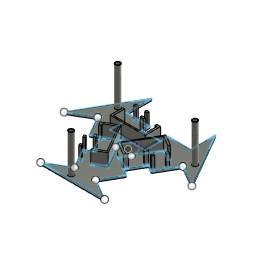
Bottom5 v3 (Autodesk Fusion 360 design; units mm, degrees)
Autodesk Fusion 360 part; units mm, degrees
sketch "草图1" plane through (0, 0, 0) normal (0, 1, 0) x (1, 0, 0)
  line L0 (0, 0) -> (6, 0)
  line L1 (6, 0) -> (6, 9.5)
  line L2 (0, 0) -> (-18.5, 0)
  line L3 (-18.5, 0) -> (-18.5, 9)
  line L4 (6, 9.5) -> (4.5, 9.5)
  line L5 (4.5, 9.5) -> (4.5, 11)
  line L6 (4.5, 11) -> (6, 11)
  line L7 (6, 11) -> (7.5, 11)
  line L8 (7.5, 11) -> (7.5, -1)
  line L9 (7.5, -1) -> (-20, -1)
  line L10 (-20, -1) -> (-20, 9)
  line L11 (-20, 9) -> (-18.5, 9)
  line L12 (-7, 11) -> (-7, 9.5)
  line L13 (-7, 9.5) -> (-4.5, 9.5)
  line L14 (-4.5, 9.5) -> (-4.5, 11)
  line L15 (-4.5, 11) -> (-7, 11)
  line L16 (-15.5, 15) -> (-17.5, 15)
  line L17 (-17.5, 15) -> (-17.5, 16.5)
  line L18 (-17.5, 16.5) -> (-15.5, 16.5)
  line L19 (-15.5, 16.5) -> (-15.5, 15)
  line L20 (-9, 15) -> (-7, 15)
  line L21 (-7, 15) -> (-7, 16.5)
  line L22 (-7, 16.5) -> (-9, 16.5)
  line L23 (-9, 16.5) -> (-9, 15)
  line L24 (4.8038, -27.3205) -> (-3.8564, -32.3205)
  line L25 (-19.3385, -9.5048) -> (-8.9462, -3.5048)
  line L26 (-17.8385, -12.1029) -> (-18.5885, -10.8038)
  line L27 (-6.0622, -10.5) -> (3.1878, -26.5215)
  line L28 (-8.9462, -3.5048) -> (4.8038, -27.3205)
  line L29 (-9.0622, -5.3038) -> (-17.2894, -10.0538)
  line L30 (-12.0394, -19.1471) -> (-13.3385, -19.8971)
  line L31 (-11.3026, -31.4234) -> (-10.3026, -33.1554)
  line L32 (-13.3385, -19.8971) -> (-12.0885, -22.0622)
  line L33 (-15.5526, -24.0622) -> (-16.8516, -24.8122)
  line L34 (3.1878, -26.5215) -> (-4.6064, -31.0215)
  line L35 (-16.8516, -24.8122) -> (-15.8516, -26.5442)
  line L36 (-15.8516, -26.5442) -> (-14.5526, -25.7942)
  line L37 (-6.0622, -10.5) -> (-9.0622, -5.3038)
  line L38 (-12.6016, -32.1734) -> (-11.3026, -31.4234)
  line L39 (-10.3026, -33.1554) -> (-11.6016, -33.9054)
  line L40 (-12.0885, -22.0622) -> (-10.7894, -21.3122)
  line L41 (-18.5885, -10.8038) -> (-19.3385, -9.5048)
  line L42 (-16.5394, -11.3529) -> (-17.8385, -12.1029)
  line L43 (-17.2894, -10.0538) -> (-16.5394, -11.3529)
  line L44 (-3.8564, -32.3205) -> (-4.6064, -31.0215)
  line L45 (-14.5526, -25.7942) -> (-15.5526, -24.0622)
  line L46 (-11.6016, -33.9054) -> (-12.6016, -32.1734)
  line L47 (-10.7894, -21.3122) -> (-12.0394, -19.1471)
  line L48 (15.1962, 7.3205) -> (23.8564, 2.3205)
  line L49 (11.8385, -22.4952) -> (1.4462, -16.4952)
  line L50 (13.3385, -19.8971) -> (12.5885, -21.1962)
  line L51 (6.0622, -10.5) -> (15.3122, 5.5215)
  line L52 (1.4462, -16.4952) -> (15.1962, 7.3205)
  line L53 (3.0622, -15.6962) -> (11.2894, -20.4462)
  line L54 (16.5394, -11.3529) -> (17.8385, -12.1029)
  line L55 (26.8026, -4.5766) -> (27.8026, -2.8446)
  line L56 (17.8385, -12.1029) -> (19.0885, -9.9378)
  line L57 (22.5526, -11.9378) -> (23.8516, -12.6878)
  line L58 (15.3122, 5.5215) -> (23.1064, 1.0215)
  line L59 (23.8516, -12.6878) -> (24.8516, -10.9558)
  line L60 (24.8516, -10.9558) -> (23.5526, -10.2058)
  line L61 (6.0622, -10.5) -> (3.0622, -15.6962)
  line L62 (28.1016, -5.3266) -> (26.8026, -4.5766)
  line L63 (27.8026, -2.8446) -> (29.1016, -3.5946)
  line L64 (19.0885, -9.9378) -> (17.7894, -9.1878)
  line L65 (12.5885, -21.1962) -> (11.8385, -22.4952)
  line L66 (12.0394, -19.1471) -> (13.3385, -19.8971)
  line L67 (11.2894, -20.4462) -> (12.0394, -19.1471)
  line L68 (23.8564, 2.3205) -> (23.1064, 1.0215)
  line L69 (23.5526, -10.2058) -> (22.5526, -11.9378)
  line L70 (29.1016, -3.5946) -> (28.1016, -5.3266)
  line L71 (17.7894, -9.1878) -> (16.5394, -11.3529)
  point P0 (0, -7)
  point P1 (-6.0622, -10.5)
  point P2 (6.0622, -10.5)
  dimension "d1" = 6
  dimension "d2" = 9.5
  dimension "d3" = 18.5
  dimension "d4" = 9
  dimension "d30" = 360
  constraint coincident L0.start L2.start
  constraint horizontal L0
  constraint perpendicular L0 L1
  constraint parallel L0 L2
  constraint perpendicular L2 L3
  constraint perpendicular L1 L4
  constraint perpendicular L4 L5
  constraint perpendicular L5 L6
  constraint perpendicular L5 L7
  constraint perpendicular L7 L8
  constraint perpendicular L8 L9
  constraint perpendicular L9 L10
  constraint perpendicular L10 L11
  constraint perpendicular L4 L12
  constraint perpendicular L12 L13
  constraint perpendicular L4 L14
  constraint perpendicular L12 L15
  constraint horizontal L16
  constraint vertical L17
  constraint horizontal L18
  constraint vertical L21
  constraint horizontal L22
  measures "d1" distance of L0.start L0.end
  measures "d2" distance of L0.end L1.end
  measures "d3" distance of L0.start L2.end
  measures "d4" distance of L2.end L3.end
sketch "草图5" plane through (0, 0, 0) normal (0, 1, 0) x (1, 0, 0)
  circle A0 centre (0, -7) radius 6
  line L0 (50, -7) -> (25, 36.3013)
  line L1 (-25, 36.3013) -> (-50, -7)
  line L2 (-25, -50.3013) -> (25, -50.3013)
  line L3 (-25, 36.3013) -> (-25, 17)
  line L4 (25, 17) -> (25, 36.3013)
  line L5 (-25, -50.3013) -> (-8.2846, -40.6506)
  line L6 (-33.2846, 2.6506) -> (-50, -7)
  line L7 (50, -7) -> (33.2846, 2.6506)
  line L8 (8.2846, -40.6506) -> (25, -50.3013)
  line L9 (-7, 17) -> (-7, 11)
  line L10 (-7, 11) -> (7.5, 11)
  line L11 (7.5, 11) -> (7.5, 17)
  line L12 (-25, 17) -> (-7, 17)
  line L13 (7.5, 17) -> (25, 17)
  line L14 (-24.5346, -12.5048) -> (-33.2846, 2.6506)
  line L15 (-19.3385, -9.5048) -> (-24.5346, -12.5048)
  line L16 (-17.2846, -25.0622) -> (-12.0885, -22.0622)
  line L17 (-8.2846, -40.6506) -> (-17.2846, -25.0622)
  line L18 (-12.0885, -22.0622) -> (-19.3385, -9.5048)
  line L19 (17.0346, -25.4952) -> (8.2846, -40.6506)
  line L20 (11.8385, -22.4952) -> (17.0346, -25.4952)
  line L21 (24.2846, -12.9378) -> (19.0885, -9.9378)
  line L22 (33.2846, 2.6506) -> (24.2846, -12.9378)
  line L23 (19.0885, -9.9378) -> (11.8385, -22.4952)
  point P0 (0, -7)
  point P1 (0, -7)
  dimension "d49" = 360
  constraint coincident P0 A0.centre
  constraint vertical L3
  constraint perpendicular L3 L12
  constraint perpendicular L4 L12
  constraint perpendicular L9 L12
  constraint perpendicular L9 L10
  constraint coincident L11.end L12
  constraint perpendicular L11 L12
  constraint collinear L12 L13
extrude "拉伸5" add sketch "草图1" along normal blind 10 makes body 1 at (-7.6667, 3.3333, -16.5) makes body 2 at (-4.3628, 3.3333, 11.4434) makes body 3 at (27.1359, 6.6667, 3.9993) makes body 4 at (24.1849, 3.3333, 12.1105) makes body 5 at (-11.9349, 3.3333, 33.3281) makes body 6 at (17.3728, 3.3333, 9.9095) makes body 7 at (-1.6667, 3.3333, 1) makes body 8 at (-11.2061, 3.3333, 20.5905) makes body 9 at (-16.1667, 3.3333, -15) makes body 10 at (-14.8859, 6.6667, 25.2169) makes body 11 at (6.0295, 6.6667, 8.5566) makes body 12 at (-6.1667, 3.3333, -9.5)
sketch "草图7" plane through (0, 0, 0) normal (0, 1, 0) x (1, 0, 0)
  circle A0 centre (-32, 17) radius 2
  circle A1 centre (-4.7846, -46.7128) radius 2
  circle A2 centre (36.7846, 8.7128) radius 2
  point P0 (0, -7)
  dimension "d34" = 360
extrude "拉伸6" add sketch "草图5" against normal blind 1.5 bodies 1 2 3 4 5 6 7 8 9 10 11 12
extrude "拉伸7" add sketch "草图7" along normal blind 30 bodies 1
hole "孔1" at (-4.7846, 30, 46.7128) direction (0, -1, 0) diameter 3 depth 10 tip angle 180 bodies 1
hole "孔2" at (-32, 30, -17) direction (0, -1, 0) diameter 3 depth 10 tip angle 180 bodies 1
hole "孔3" at (36.7846, 30, -8.7128) direction (0, -1, 0) diameter 3 depth 10 tip angle 180 bodies 1
pattern_circular "C-阵列1" [suppressed]
extrude "拉伸2" [suppressed]
extrude "拉伸3" [suppressed]
copy_body "实体->零部件1" [suppressed] in component "Component"
copy_body "实体->零部件2" [suppressed] in component "Component'"
copy_body "实体->零部件3" [suppressed] in component "Component''"
copy_body "实体->零部件4" [suppressed] in component "Component'''"
sketch "草图3" plane through (0, 0, 0) normal (0, 1, 0) x (1, 0, 0)
  circle A0 centre (0, -7) radius 6
  circle A1 centre (0, -7) radius 50
  constraint concentric A0 A1
boxprimitive "长方体基本要素1" [suppressed]
